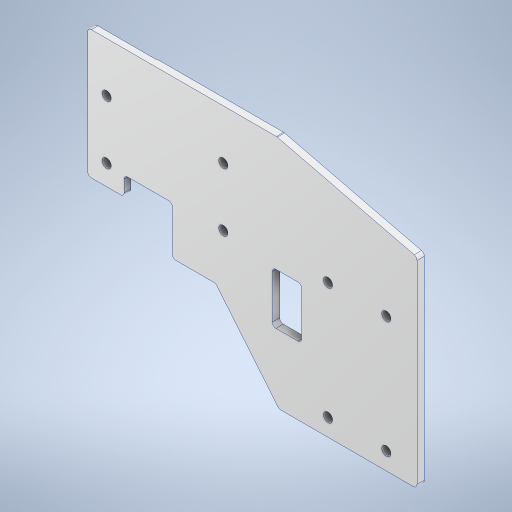
# Autodesk Inventor part: connectplate2
Saved by Autodesk Inventor 2024 (Build 280153000, 153)
## iProperties
Created: 2025-06-26
Part Number: connectplate2
Material: アルミニウム 6061
Document SubType Name: Sheet Metal
Designer: kshau
Density: 2.7 g/cm^3
Appearance: アルミニウム - フラット
Sheet Metal Rule: Default
Author: kshau
Autodesk Inventor part; units mm, degrees
ref_plane "YZ Plane" through (0, 0, 0) normal (1, 0, 0) x (0, 1, 0)
ref_plane "XZ Plane" through (0, 0, 0) normal (0, 1, 0) x (-1, 0, 0)
ref_plane "XY Plane" through (0, 0, 0) normal (0, 0, 1) x (1, 0, 0)
sketch "スケッチ1" plane through (0, 0, 0) normal (0, 0, 1) x (1, 0, 0)
  line L0 (0, 0) -> (-90.3, 0)
  line L1 (-90.3, 0) -> (-90.3, 64.35)
  line L2 (-90.3, 64.35) -> (0, 64.35)
  line L3 (0, 64.35) -> (0, 0)
  line L4 (-90.3, 21.15) -> (0, 21.15)
  line L5 (-55.219, 21.15) -> (-37.813, 0)
  line L6 (-90.3, 29.15) -> (0, 29.15)
  line L7 (-80.3, 29.15) -> (-67.1, 29.15)
  line L8 (-67.1, 29.15) -> (-67.1, 34.35)
  line L9 (-67.1, 34.35) -> (-80.3, 34.35)
  line L10 (-80.3, 34.35) -> (-80.3, 29.15)
  line L11 (-67.1, 29.15) -> (-67.1, 21.15)
  line L12 (-38.44, 64.35) -> (0, 54.9793)
  dimension "d0" = 90.3
  dimension "d1" = 64.35
  dimension "d2" = 21.15
  dimension "d3" = 55.219
  dimension "d4" = 37.813
  dimension "d5" = 35.2
  dimension "d6" = 10
  dimension "d7" = 5.2
  dimension "d8" = 13.2
  dimension "d9" = 166.3
  dimension "d10" = 51.86
  constraints: 26 end point, 10 point on line, 5 perpendicular, 4 parallel, 2 horizontal
  measures "d0" distance of L1.end L2.end
  measures "d1" distance of L2.end L0.start
  measures "d2" distance between parallel lines of L0 L4
  measures "d3" distance from line of L3 L5.start
  measures "d4" distance from line of L3 L5.end
  measures "d5" distance between parallel lines of L2 L6
  measures "d6" distance between parallel lines of L1 L10
  measures "d7" distance between parallel lines of L6 L9
  measures "d8" distance of L8.end L9.end
  measures "d9" angle of L2 L12
  measures "d10" distance from line of L1 L12.start
extrude "押し出し1" add sketch "スケッチ1" along normal blind 2 contours L0 L5 L4 L3 | L4 L11 L6 L3 | L6 L8 L9 L10 L1 L2 L12 L3
sketch "スケッチ2" plane through (0, 0, 2) normal (0, 0, 1) x (1, 0, 0)
  line L0 (-85.1, 34.75) -> (-53.1, 34.75)
  line L1 (-53.1, 34.75) -> (-53.1, 50.75)
  line L2 (-53.1, 50.75) -> (-85.1, 50.75)
  line L3 (-85.1, 50.75) -> (-85.1, 34.75)
  line L4 (-90.3, 29.15) -> (-80.3, 29.15) projected
  line L5 (-90.3, 64.35) -> (-90.3, 29.15) projected
  line L6 (-8.4, 4.75) -> (-24.4, 4.75)
  line L7 (-24.4, 4.75) -> (-24.4, 36.75)
  line L8 (-24.4, 36.75) -> (-8.4, 36.75)
  line L9 (-8.4, 36.75) -> (-8.4, 4.75)
  line L10 (0, 0) -> (0, 54.9793) projected
  line L11 (-37.813, 0) -> (0, 0) projected
  dimension "d13" = 5.6
  dimension "d14" = 5.2
  dimension "d15" = 16
  dimension "d16" = 32
  dimension "d17" = 8.4
  dimension "d18" = 4.75
  dimension "d19" = 16
  dimension "d20" = 32
  constraints: 16 end point, 8 coincident, 4 parallel, 2 horizontal, 2 perpendicular
  measures "d13" distance between parallel lines of L4 L0
  measures "d14" distance between parallel lines of L5 L3
  measures "d15" distance of L2.end L0.start
  measures "d16" distance of L1.end L2.end
  measures "d17" distance between parallel lines of L10 L9
  measures "d18" distance between parallel lines of L11 L6
  measures "d19" distance of L7.end L8.end
  measures "d20" distance of L6.end L7.end
hole "穴1" at (-85.1, 50.75, 2) at (-85.1, 34.75, 2) at (-53.1, 34.75, 2) at (-53.1, 50.75, 2) at (-24.4, 4.75, 2) at (-8.4, 4.75, 2) at (-8.4, 36.75, 2) at (-24.4, 36.75, 2) direction (0, 0, -1) diameter 2.5 end through all
fillet "フィレット1" radius 1 11 edges at (0, 0, 1) (0, 54.9793, 1) (-90.3, 64.35, 1) (-90.3, 29.15, 1) (-80.3, 29.15, 1) (-80.3, 34.35, 1) (-67.1, 34.35, 1) (-67.1, 21.15, 1) (-55.219, 21.15, 1) (-37.813, 0, 1) (-38.44, 64.35, 1)
sketch "スケッチ3" plane through (0, 0, 0) normal (0, 0, -1) x (-1, 0, 0)
  line L0 (31.65, 18.75) -> (39.65, 18.75)
  line L1 (39.65, 18.75) -> (39.65, 32.75)
  line L2 (39.65, 32.75) -> (31.65, 32.75)
  line L3 (31.65, 32.75) -> (31.65, 18.75)
  circle A0 centre (24.4, 4.75) radius 1.25 projected
  circle A1 centre (24.4, 36.75) radius 1.25 projected
  point P0 (0, 0)
  dimension "d29" = 14
  dimension "d30" = 14
  dimension "d31" = 8
  dimension "d32" = 6
  constraints: 8 end point, 2 parallel, 1 horizontal, 1 perpendicular
  measures "d29" distance from line of A0.centre L0
  measures "d30" distance of L2.end L0.start
  measures "d31" distance of L1.end L2.end
  measures "d32" distance edge to line of A1 L3
extrude "押し出し2" cut sketch "スケッチ3" against normal blind 10 contours L3 L2 L1 L0
fillet "フィレット2" radius 1 4 edges at (-31.65, 18.75, 1) (-31.65, 32.75, 1) (-39.65, 32.75, 1) (-39.65, 18.75, 1)
sketch "スケッチ5" plane through (0, 0, 0) normal (0, 0, -1) x (-1, 0, 0)
  line L0 (79.3, 34.35) -> (68.1, 34.35) projected
  line L1 (73.3, 34.35) -> (73.3, 64.35)
  line L2 (38.5601, 64.35) -> (89.3, 64.35) projected
  line L3 (90.3, 63.35) -> (90.3, 30.15) projected
  arc A0 (80.3, 33.35) -> (79.3, 34.35) centre (79.3, 33.35) ccw projected
  arc A1 (80.3, 33.35) -> (79.3, 34.35) centre (79.3, 33.35) ccw
  arc A2 (80.3, 30.15) -> (81.3, 29.15) centre (81.3, 30.15) ccw projected
  arc A3 (80.3, 30.15) -> (81.3, 29.15) centre (81.3, 30.15) ccw
  arc A4 (89.3, 29.15) -> (90.3, 30.15) centre (89.3, 30.15) ccw projected
  arc A5 (89.3, 29.15) -> (90.3, 30.15) centre (89.3, 30.15) ccw
  arc A6 (90.3, 63.35) -> (89.3, 64.35) centre (89.3, 63.35) ccw projected
  arc A7 (90.3, 63.35) -> (89.3, 64.35) centre (89.3, 63.35) ccw
  line L4 (73.3, 64.35) -> (89.3, 64.35)
  line L5 (90.3, 63.35) -> (90.3, 30.15)
  line L6 (89.3, 29.15) -> (81.3, 29.15)
  line L7 (80.3, 30.15) -> (80.3, 33.35)
  line L8 (79.3, 34.35) -> (73.3, 34.35)
  point P0 (0, 0)
  dimension "d36" = 17
  constraints: 12 end point, 8 point on circle, 4 centre point, 3 perpendicular, 2 collinear, 2 point on line, 1 tangent, 1 vertical
  measures "d36" distance between parallel lines of L3 L1
extrude "押し出し3" cut sketch "スケッチ5" against normal blind 0.19
equation "\"BendRadius\" = Thickness"
equation "\"BendReliefWidth\" = Thickness"
equation "\"BendReliefDepth\" = 0.5 * Thickness"
equation "\"CornerReliefSize\" = 4 * Thickness"
equation "\"MinimumRemnant\" = 2 * Thickness"
equation "\"TransitionRadius\" = BendRadius"
equation "\"JacobiRadiusSize\" = BendRadius"
equation "\"GapSize\" = Thickness"
equation "\"Thickness\" = 3.048"
